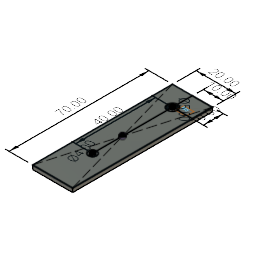
kobra_s1_bed_supports (Autodesk Fusion 360 design; units mm, degrees)
Autodesk Fusion 360 part; units mm, degrees
sketch "Sketch1" plane through (0, 0, 0) normal (0, 0, 1) x (1, 0, 0)
  line L0 (10, -35) -> (-10, -35)
  line L1 (-10, -35) -> (-10, 35)
  line L2 (-10, 35) -> (10, 35)
  line L3 (10, 35) -> (10, -35)
  line L4 (10, -35) -> (-10, 35) construction
  line L5 (-10, -35) -> (10, 35) construction
  line L6 (10, 35) -> (0, 35)
  line L7 (0, 35) -> (0, 25)
  line L8 (0, 25) -> (10, 25)
  line L9 (10, 25) -> (10, 35)
  line L10 (0, 25) -> (0, -15)
  circle A0 centre (0, -15) radius 2
  circle A1 centre (0, 25) radius 2.5
  dimension "d1" = 20
  dimension "d2" = 70
  dimension "d3" = 10
  dimension "d4" = 10
  dimension "d5" = 40
  dimension "d25" = 4
  dimension "d26" = 5
  constraint horizontal L0
  constraint perpendicular L0 L1
  constraint parallel L0 L2
  constraint parallel L1 L3
  constraint coincident L4 origin
  constraint coincident L5 origin
  constraint horizontal L6
  constraint vertical L7
  constraint horizontal L8
  constraint vertical L9
  constraint perpendicular L8 L10
  constraint coincident L10.end A0.centre
  constraint coincident L7.end L8.start
  measures "d1" distance of L1.end L2.end
  measures "d2" distance of L0.end L1.end
  measures "d3" distance of L2.end L6.end
  measures "d4" distance of L2.end L8.end
  measures "d5" distance of L7.end L10.end
  measures "d25" diameter of A0
  measures "d26" diameter of A1
extrude "Extrude1" add sketch "Sketch1" against normal blind 2 contours L0 L1 L2 L3 L7 L8 A1 | L2 L3 L6 L7 L8 L9 A1 | L8 L10 A1 | L7 L8 A1 | L7 L10 A1 | A0
hole "Hole1" at (0, 25, 0) direction (0, 0, -1) diameter 4.234 depth 3 tip angle 118
thread "Thread1" "ISO Metric profile 5.0 M5x0.8 M5x0.8 6H" major diameter 5.12 minor diameter 4.234 pitch 0.8 angle 60 modelled right hand crest width 0.2219 on face at (0.2108, 22.8935, -1.3333) crest through (2.117, 25, -0.2)
sketch "Sketch2" plane through (0, 0, 0) normal (0, 0, 1) x (1, 0, 0)
  line L0 (2.2126, 24.4763) -> (7.2126, 24.4763) construction
  line L1 (7.2126, 24.4763) -> (7.2126, 28.4763) construction
  line L2 (7.2126, 28.4763) -> (2.2126, 28.4763) construction
  line L3 (2.2126, 28.4763) -> (2.2126, 24.4763) construction
  dimension "d18" = 2
  dimension "d19" = 0
hole "Hole3" at (0, -15, 0) direction (0, 0, -1) diameter 4 depth 20 tip angle 118
equation "d19 = 'M5'"
